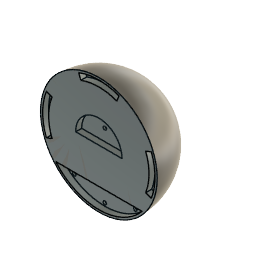
Abstract_Embodiment (Autodesk Fusion 360 design; units mm, degrees)
Autodesk Fusion 360 part; units mm, degrees
sketch "Sketch1" plane through (0, 0, 0) normal (0, 0, 1) x (1, 0, 0)
  line L0 (0, 0) -> (102, 0)
  line L1 (0, 0) -> (0, 102)
  arc A0 (102, 0) -> (0, 102) centre (0, 0) ccw
  dimension "d1" = 204
  constraint coincident L0.start L1.start
  constraint horizontal L0
  constraint perpendicular L0 L1
  measures "d1" diameter of A0
revolve "Revolve1" add sketch "Sketch1" angle 360 about axis through (0, 0, 0) along (0, 1, 0)
sketch "Sketch2" plane through (0, 0, 0) normal (0, -1, 0) x (1, 0, 0)
  circle A0 centre (0, 0) radius 102
  line L0 (0, 0) -> (0, -0.5) construction
  line L1 (0, -0.5) -> (-40.4969, -0.5) construction
  line L2 (-40.4969, -0.5) -> (40.4969, -0.5)
  arc A1 (40.4969, -0.5) -> (-40.4969, -0.5) centre (0, 0) ccw
  dimension "d3" = 81
  dimension "d4" = 0.5
  constraint coincident A0.centre L0.start
  constraint vertical L0
  constraint perpendicular L0 L1
  measures "d3" diameter of A1
  measures "d4" distance of A0.centre L0.end
extrude "Extrude1" cut sketch "Sketch2" against normal blind 10.5 contours L2 A1
sketch "Sketch3" plane through (0, 0, 0) normal (0, -1, 0) x (1, 0, 0)
  line L0 (40.4969, -0.5) -> (-40.4969, -0.5)
  arc A0 (40.4969, -0.5) -> (-40.4969, -0.5) centre (0, 0) ccw
  circle A1 centre (0, 0) radius 102
sketch "Sketch4" plane through (0, 0, 0) normal (0, -1, 0) x (1, 0, 0)
  line L0 (0, 0) -> (0, -64) construction
  line L1 (40, -64) -> (40, -63)
  line L2 (40, -46.5) -> (-40, -81.5) construction
  line L3 (-40, -46.5) -> (0, -64) construction
  line L4 (0, -64) -> (0, -63)
  line L5 (0, -63) -> (-61.0824, -63)
  line L6 (0, -63) -> (61.0824, -63)
  line L7 (-40, -63) -> (-40, -64)
  arc A0 (-36.3095, -79.8854) -> (-32.524, -81.5) centre (0, 0) ccw
  line L8 (31.4468, 81.9217) -> (35.2097, 91.7243)
  line L9 (0, 0) -> (98.25, 0) construction
  line L10 (-31.4468, 81.9217) -> (-35.2097, 91.7243)
  line L11 (0, 0) -> (98.25, 0) construction
  line L12 (81.9217, 31.4468) -> (91.7243, 35.2097)
  line L13 (0, 0) -> (98.25, 0) construction
  line L14 (81.9217, -31.4468) -> (91.7243, -35.2097)
  line L15 (0, 0) -> (98.25, 0) construction
  line L16 (0, 114.2451) -> (0, -120) construction
  line L17 (-81.9217, 31.4468) -> (-91.7243, 35.2097)
  line L18 (-81.9217, -31.4468) -> (-91.7243, -35.2097)
  arc A1 (-81.9217, 31.4468) -> (-81.9217, -31.4468) centre (0, 0) ccw
  arc A2 (81.9217, -31.4468) -> (81.9217, 31.4468) centre (0, 0) ccw
  arc A3 (31.4468, 81.9217) -> (-31.4468, 81.9217) centre (0, 0) ccw
  arc A4 (35.2097, 91.7243) -> (-35.2097, 91.7243) centre (0, 0) ccw
  line L19 (-61.0824, -63) -> (-75.3927, -63)
  line L20 (61.0824, -63) -> (75.3927, -63)
  arc A5 (-91.7243, 35.2097) -> (-91.7243, -35.2097) centre (0, 0) ccw
  arc A6 (-75.3927, -63) -> (75.3927, -63) centre (0, 0) ccw
  arc A7 (91.7243, -35.2097) -> (91.7243, 35.2097) centre (0, 0) ccw
  point P0 (0, -64)
  dimension "d9" = 196.5
  dimension "d10" = 175.5
  dimension "d11" = 64
  dimension "d13" = 35
  dimension "d14" = 1
  dimension "d15" = 69
  dimension "d16" = 111
  dimension "d17" = 21
  dimension "d18" = 21
  constraint coincident L0.start A0.centre
  constraint concentric A2 A7
  constraint vertical L0
  constraint parallel L1 L7
  constraint coincident L2 P0
  constraint coincident L3 P0
  constraint coincident P0 L0.end
  constraint vertical L4
  constraint perpendicular L5 L7
  constraint perpendicular L1 L6
  constraint coincident L5 L7.start
  constraint coincident L6 L1.end
  constraint coincident L2 A0.start
  constraint concentric A0 A1
  constraint horizontal L9
  constraint horizontal L11
  constraint horizontal L13
  constraint horizontal L15
  constraint parallel L0 L16
  constraint symmetric L12.end L16 L17.end
  constraint symmetric L14.end L16 L18.end
  constraint concentric A1 A3
  constraint concentric A2 A3
  constraint concentric A4 A7
  constraint parallel L5 L19
  constraint parallel L6 L20
  constraint concentric A5 A6
  constraint concentric A6 A7
  measures "d9" diameter of A5
  measures "d10" diameter of A0
  measures "d11" distance of L0.start P0
  measures "d13" distance of L3.start L2.end
  measures "d14" distance of P0 L4.end
  measures "d15" angle of L8 L9
  measures "d16" angle of L10 L11
  measures "d17" angle of L12 L13
  measures "d18" angle of L14 L15
extrude "Extrude2" cut sketch "Sketch4" against normal blind 10.5
sketch "Sketch5" plane through (0, 0, 0) normal (0, -1, 0) x (1, 0, 0)
  circle A0 centre (0, 0) radius 93 construction
  line L0 (0, 0) -> (-16.1493, 91.5871) construction
  line L1 (0, 0) -> (93, 0) construction
  line L2 (0, 0) -> (16.1493, 91.5871) construction
  line L3 (0, 0) -> (93, 0) construction
  line L4 (0, 0) -> (-91.5871, 16.1493) construction
  line L5 (0, 0) -> (93, 0) construction
  line L6 (0, 0) -> (-91.5871, -16.1493) construction
  line L7 (0, 0) -> (93, 0) construction
  line L8 (0, 0) -> (91.5871, 16.1493) construction
  line L9 (0, 0) -> (93, 0) construction
  line L10 (0, 0) -> (91.5871, -16.1493) construction
  line L11 (0, 0) -> (93, 0) construction
  line L12 (0, 0) -> (0, -93) construction
  line L13 (0, 0) -> (-53.3426, -76.1811) construction
  line L14 (0, 0) -> (93, 0) construction
  line L15 (0, 0) -> (53.3426, -76.1811) construction
  circle A1 centre (0, 0) radius 20 construction
  line L16 (0, 0) -> (0, 20) construction
  circle A2 centre (-16.1493, 91.5871) radius 3
  circle A3 centre (16.1493, 91.5871) radius 3
  line L17 (0, 130) -> (0, -112.7435) construction
  circle A4 centre (-91.5871, 16.1493) radius 3
  circle A5 centre (-91.5871, -16.1493) radius 3
  circle A6 centre (-53.3426, -76.1811) radius 3
  circle A7 centre (91.5871, 16.1493) radius 3
  circle A8 centre (91.5871, -16.1493) radius 3
  circle A9 centre (53.3426, -76.1811) radius 3
  circle A10 centre (0, 20) radius 3
  circle A11 centre (0, -93) radius 3
  dimension "d21" = 186
  dimension "d22" = 100
  dimension "d23" = 80
  dimension "d24" = 170
  dimension "d25" = 170
  dimension "d26" = 10
  dimension "d27" = 10
  dimension "d28" = 125
  dimension "d29" = 40
  dimension "d30" = 6
  dimension "d31" = 6
  dimension "d32" = 6
  dimension "d33" = 6
  dimension "d34" = 6
  dimension "d35" = 6
  dimension "d36" = 6
  constraint coincident A0.centre L0.start
  constraint horizontal L1
  constraint horizontal L3
  constraint horizontal L5
  constraint horizontal L7
  constraint horizontal L9
  constraint horizontal L11
  constraint coincident A0 L12.end
  constraint perpendicular L3 L12
  constraint horizontal L14
  constraint symmetric A0.centre L12 L0.start
  constraint symmetric L12 L13.end L15.end
  constraint coincident A1 L16.end
  constraint vertical L16
  constraint coincident L0.end A2.centre
  constraint coincident L2.end A3.centre
  constraint parallel L12 L17
  constraint coincident L4.end A4.centre
  constraint coincident L6.end A5.centre
  constraint coincident L13.end A6.centre
  constraint symmetric L17 A4 A7
  constraint symmetric L17 A5 A8
  constraint symmetric L17 A6 A9
  constraint coincident L16.end A10.centre
  constraint coincident L12.end A11.centre
  measures "d21" diameter of A0
  measures "d22" angle of L0 L1
  measures "d23" angle of L2 L3
  measures "d24" angle of L4 L5
  measures "d25" angle of L6 L7
  measures "d26" angle of L8 L9
  measures "d27" angle of L10 L11
  measures "d28" angle of L13 L14
  measures "d29" diameter of A1
  measures "d30" diameter of A2
  measures "d31" diameter of A3
  measures "d32" diameter of A4
  measures "d33" diameter of A5
  measures "d34" diameter of A6
  measures "d35" diameter of A10
  measures "d36" diameter of A11
extrude "Extrude3" cut sketch "Sketch5" against normal blind 13.7
